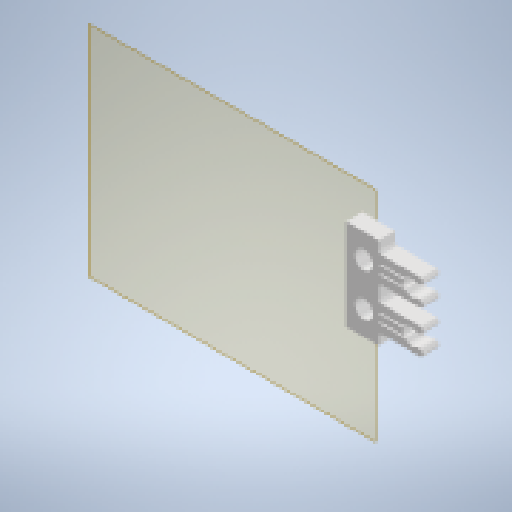
# Autodesk Inventor part: Fuse holdere
Saved by Autodesk Inventor 2024 (Build 280153000, 153)
## iProperties
Created: 2024-03-29
Part Number: Fuse holdere
Material: Generic
Document SubType Name: Modeling
Designer: jens1
Density: 1 g/cm^3
Appearance: Default
Author: jens1
Autodesk Inventor part; units mm, degrees
ref_plane "YZ Plane" through (0, 0, 0) normal (1, 0, 0) x (0, 1, 0)
ref_plane "XZ Plane" through (0, 0, 0) normal (0, 1, 0) x (-1, 0, 0)
ref_plane "XY Plane" through (0, 0, 0) normal (0, 0, 1) x (1, 0, 0)
ref_plane "Work Plane1" through (373.0741, 421.919, 355.2069) normal (0, 0, 1) x (1, 0, 0)
sketch "Sketch1" plane through (373.0741, 421.919, 355.2069) normal (0, 0, 1) x (1, 0, 0)
  line L0 (-40, 30.5) -> (-40, -30.5) projected
  line L1 (-40, -30.5) -> (45, -30.5) projected
  circle A0 centre (5.1305, -24.4679) radius 3.2 projected
  circle A1 centre (-24.4679, -5.1305) radius 3.2 projected
  circle A2 centre (-5.1305, 24.4679) radius 3.2 projected
  circle A3 centre (24.4679, 5.1305) radius 3.2 projected
  circle A4 centre (0, 0) radius 16.75 projected
  line L2 (40, 25.5) -> (50, 25.5)
  line L3 (50, 25.5) -> (50, -25.5)
  line L4 (50, -25.5) -> (40, -25.5)
  line L5 (40, -25.5) -> (40, 25.5)
  circle A5 centre (60, 18) radius 2.25
  circle A6 centre (60, 18) radius 2.5
  line L6 (50, 19) -> (57.7087, 19)
  line L7 (57.7087, 19) -> (57.7087, 17)
  line L8 (57.7087, 17) -> (50, 17)
  line L9 (50, 17) -> (50, 19)
  line L10 (50, 19.5) -> (58.3229, 19.5)
  line L11 (57.7087, 18) -> (50, 18)
  line L12 (58.3229, 16.5) -> (50, 16.5)
  line L13 (62.6125, 22) -> (50, 22)
  line L14 (50, 14) -> (62.6125, 14)
  line L15 (63.5021, 20.5433) -> (62.2478, 18.1)
  line L16 (63.5021, 15.4567) -> (62.2478, 17.9)
  arc A7 (63.5021, 20.5433) -> (62.6125, 22) centre (62.6125, 21) ccw
  arc A8 (62.6125, 14) -> (63.5021, 15.4567) centre (62.6125, 15) ccw
  line L17 (50, 11.5) -> (40, 11.5)
  circle A9 centre (60, 5) radius 2.25
  circle A10 centre (60, 5) radius 2.5
  line L18 (50, 4) -> (57.7087, 4)
  line L19 (57.7087, 6) -> (50, 6)
  line L20 (50, 3.5) -> (58.3229, 3.5)
  line L21 (58.3229, 6.5) -> (50, 6.5)
  line L22 (62.6125, 1) -> (50, 1)
  line L23 (50, 9) -> (62.6125, 9)
  line L24 (63.5021, 2.4567) -> (62.2478, 4.9)
  line L25 (63.5021, 7.5433) -> (62.2478, 5.1)
  arc A11 (62.6125, 1) -> (63.5021, 2.4567) centre (62.6125, 2) ccw
  arc A12 (63.5021, 7.5433) -> (62.6125, 9) centre (62.6125, 8) ccw
  line L26 (40, 25.5) -> (50, 25.5)
  line L27 (50, 25.5) -> (50, -2.5)
  line L28 (50, -2.5) -> (40, -2.5)
  line L29 (40, -2.5) -> (40, 25.5)
  circle A13 centre (45.3451, 5) radius 2.5 projected
  circle A14 centre (45, -8) radius 2.5 projected
  circle A15 centre (45.3451, 18) radius 2.5 projected
  circle A16 centre (45, -21) radius 2.5 projected
  arc A17 (45, -30.5) -> (50, -25.5) centre (45, -25.5) ccw projected
  line L30 (50, 25.5) -> (50, -25.5) projected
  arc A18 (50, 25.5) -> (45, 30.5) centre (45, 25.5) ccw projected
  line L31 (-40, 30.5) -> (45, 30.5) projected
  point P0 (-373.0741, -421.919)
  point P1 (40, 30.5)
  point P2 (53.8544, 18)
  point P3 (64.25, 22)
  point P4 (64.25, 14)
  point P5 (50, 1)
  point P6 (62.2478, 4.9)
  point P7 (50, 3.5)
  point P8 (50, 4)
  point P9 (50, 6)
  point P10 (50, 6.5)
  point P11 (50, 9)
  point P12 (50, 17)
  point P13 (62.2478, 18.1)
  point P14 (40, -2.5)
  point P15 (62.4505, 17.5051)
  point P16 (58, 16.5)
  point P17 (50, 16.5)
  point P18 (50, 14)
  point P19 (50, 22)
  point P20 (50, 19.5)
  point P21 (58, 19.5)
  point P22 (62.4505, 18.4949)
  point P23 (50, 9)
  point P24 (50, 6.5)
  point P25 (58, 6.5)
  point P26 (62.4505, 5.4949)
  point P27 (50, 17)
  point P28 (50, 19)
  point P29 (62.4505, 4.5051)
  point P30 (58, 3.5)
  point P31 (50, 3.5)
  point P32 (50, 1)
  point P33 (50, 6)
  point P34 (50, 4)
  point P35 (40, -2.5)
  dimension "d1" = 5
  dimension "d4" = 4.5
  dimension "d5" = 5
  dimension "d6" = 10
  dimension "d7" = 2
  dimension "d8" = 1
  dimension "d9" = 1.5
  dimension "d10" = 1.5
  dimension "d11" = 2.5
  dimension "d12" = 2.5
  dimension "d13" = 14.25
  dimension "d14" = 14.25
  dimension "d15" = 0.2
  dimension "d16" = 0
  dimension "d17" = 0.1
  dimension "d18" = 1
  dimension "d19" = 3.5
  dimension "d20" = 6.5
  dimension "d21" = 3.5
  constraints: 54 end point, 20 symmetric about line, 18 point on circle, 11 parallel, 8 centre point, 5 point on line, 4 horizontal, 4 tangent, 3 midpoint, 2 coincident, 2 perpendicular, 1 equal radius, 1 vertical, 15 other
  measures "d1" distance between parallel lines of L1 L4
  measures "d4" diameter of A5
  measures "d5" diameter of A6
  measures "d7" distance of L6.end L7.end
  measures "d8" distance between parallel lines of L8 L11
  measures "d9" distance from line of L10 point (53.854, 18)
  measures "d10" distance between parallel lines of L12 L11
  measures "d11" distance between parallel lines of L10 L13
  measures "d12" distance between parallel lines of L12 L14
  measures "d13" distance of point (64.25, 22) L13.end
  measures "d14" distance of L14.start point (64.25, 14)
  measures "d15" distance of L16.end L15.end
  measures "d16" horizontal distance of L15.end L16.end
  measures "d17" vertical distance of A5.centre L16.end
  measures "d18" radius of A7
  measures "d19" distance between parallel lines of L2 L13
  measures "d20" distance from line of A5.centre L17
  measures "d21" distance between parallel lines of L22 L28
extrude "Extrusion1" add sketch "Sketch1" along normal blind 5 contours L3 L17 L5 L2 | L13 A7 L15 A6 L10 L3 | L28 L5 L17 L3 | L3 L20 A10 L24 A11 L22 | L6 A6 L11 L3 | L3 L12 A6 L16 A8 L14 | L23 A12 L25 A10 L21 L3 | L11 A6 L8 L3 | L3 L19 A10 L18 | A13 | A15
fillet "Fillet1" radius 2 4 edges at (435.5246, 440.414, 357.7069) (435.5246, 439.4241, 357.7069) (435.5246, 427.414, 357.7069) (435.5246, 426.4241, 357.7069)
fillet "Fillet2" radius 1 8 edges at (423.0741, 441.419, 357.7069) (423.0741, 438.419, 357.7069) (423.0741, 443.919, 357.7069) (423.0741, 435.919, 357.7069) (423.0741, 430.919, 357.7069) (423.0741, 428.419, 357.7069) (423.0741, 425.419, 357.7069) (423.0741, 422.919, 357.7069)
sketch "Sketch2" plane through (373.0741, 421.919, 360.2069) normal (0, 0, 1) x (1, 0, 0)
  line L0 (58, 3.5) -> (50.866, 3.5) projected
  line L1 (50, 4) -> (57.7087, 4) projected
  arc A0 (57.7087, 6) -> (57.7087, 4) centre (60, 5) ccw projected
  line L2 (57.7087, 6) -> (50, 6) projected
  line L3 (50.866, 6.5) -> (58, 6.5) projected
  arc A1 (63.5021, 7.5433) -> (62.6125, 9) centre (62.6125, 8) ccw projected
  line L4 (62.6125, 9) -> (51, 9) projected
  line L5 (50, 10) -> (50, 13) projected
  line L6 (51, 14) -> (62.6125, 14) projected
  arc A2 (62.6125, 14) -> (63.5021, 15.4567) centre (62.6125, 15) ccw projected
  line L7 (58, 16.5) -> (50.866, 16.5) projected
  line L8 (50, 17) -> (57.7087, 17) projected
  arc A3 (57.7087, 19) -> (57.7087, 17) centre (60, 18) ccw projected
  line L9 (57.7087, 19) -> (50, 19) projected
  line L10 (50.866, 19.5) -> (58, 19.5) projected
  arc A4 (63.5021, 20.5433) -> (62.6125, 22) centre (62.6125, 21) ccw projected
  line L11 (62.6125, 22) -> (51, 22) projected
  line L12 (50, 25.5) -> (40, 25.5) projected
  line L13 (51, 1) -> (62.6125, 1) projected
  arc A5 (62.6125, 1) -> (63.5021, 2.4567) centre (62.6125, 2) ccw projected
  arc A6 (58, 3.5) -> (61.1705, 2.791) centre (60, 5) ccw projected
  arc A7 (61.1705, 7.209) -> (58, 6.5) centre (60, 5) ccw projected
  arc A8 (58, 16.5) -> (61.1705, 15.791) centre (60, 18) ccw projected
  arc A9 (61.1705, 20.209) -> (58, 19.5) centre (60, 18) ccw projected
  line L14 (40, 25.5) -> (40, -2.5) projected
  arc A10 (50, 10) -> (51, 9) centre (51, 10) ccw projected
  arc A11 (51, 14) -> (50, 13) centre (51, 13) ccw projected
  arc A12 (50, 17) -> (50.866, 16.5) centre (50.866, 17.5) ccw projected
  arc A13 (50.866, 19.5) -> (50, 19) centre (50.866, 18.5) ccw projected
  arc A14 (50, 23) -> (51, 22) centre (51, 23) ccw projected
  line L15 (50, 23) -> (50, 25.5) projected
  line L16 (40, -2.5) -> (50, -2.5) projected
  line L17 (50, -2.5) -> (50, 0) projected
  arc A15 (51, 1) -> (50, 0) centre (51, 0) ccw projected
  arc A16 (50, 4) -> (50.866, 3.5) centre (50.866, 4.5) ccw projected
  arc A17 (50.866, 6.5) -> (50, 6) centre (50.866, 5.5) ccw projected
  arc A18 (63.5021, 2.4567) -> (61.1705, 2.791) centre (62.107, 1.0237) ccw projected
  arc A19 (61.1705, 7.209) -> (63.5021, 7.5433) centre (62.107, 8.9763) ccw projected
  arc A20 (63.5021, 15.4567) -> (61.1705, 15.791) centre (62.107, 14.0237) ccw projected
  arc A21 (61.1705, 20.209) -> (63.5021, 20.5433) centre (62.107, 21.9763) ccw projected
  point P0 (-373.0741, -421.919)
  point P1 (45.3451, 18)
  point P2 (45.3451, 5)
  dimension "d26" = 0
  dimension "d27" = 13
  dimension "d28" = 7.5
  measures "d26" horizontal distance of point (45.345, 5) point (45.345, 18)
  measures "d27" distance of point (45.345, 18) point (45.345, 5)
  measures "d28" distance from line of L12 point (45.345, 18)
hole "Hole1" at (418.4192, 439.919, 360.2069) at (418.4192, 426.919, 360.2069) direction (0, 0, -1) diameter 5.5 end through all
sketch "Sketch3" plane through (373.0741, 421.919, 355.2069) normal (0, 0, 1) x (1, 0, 0)
  line L0 (68.3936, 26.3924) -> (78.3936, 26.3924)
  line L1 (78.3936, 26.3924) -> (78.3936, -1.6076)
  line L2 (78.3936, -1.6076) -> (68.3936, -1.6076)
  line L3 (68.3936, -1.6076) -> (68.3936, 26.3924)
  line L4 (78.3936, 26.3924) -> (68.3936, 26.3924)
  line L5 (68.3936, 26.3924) -> (68.3936, 12.3924)
  line L6 (68.3936, 12.3924) -> (78.3936, 12.3924)
  line L7 (78.3936, 12.3924) -> (78.3936, 26.3924)
  line L8 (92.6436, 14.3924) -> (78.3936, 14.3924)
  line L9 (78.3936, 14.3924) -> (78.3936, 14.5958)
  line L10 (78.3936, 19.3924) -> (86.1023, 19.3924)
  line L11 (86.1023, 19.3924) -> (86.1023, 17.3924)
  line L12 (86.1023, 17.3924) -> (78.3936, 17.3924)
  line L13 (78.3936, 17.3924) -> (78.3936, 19.3924)
  circle A0 centre (88.3936, 18.3924) radius 2.25
  circle A1 centre (88.3936, 18.3924) radius 2.5
  line L14 (91.6425, 23.6467) -> (90.6413, 18.4924)
  line L15 (92.6436, 14.3924) -> (90.6413, 18.2924)
  line L16 (78.3936, 16.8924) -> (86.3936, 16.8924)
  line L17 (78.1639, 19.8924) -> (86.3936, 19.8924)
  line L18 (78.3936, 23.6467) -> (91.6425, 23.6467)
  point P0 (-373.0741, -421.919)
  point P1 (73.3936, 26.3924)
  point P2 (82.2479, 17.3924)
  dimension "d36" = 10
  dimension "d37" = 28
  dimension "d38" = 14
  dimension "d44" = 2
  dimension "d45" = 4.5
  dimension "d46" = 5
  dimension "d47" = 1
  dimension "d48" = 10
  dimension "d49" = 0.2
  dimension "d50" = 0.1
  dimension "d51" = 14.25
  dimension "d53" = 2.5
  dimension "d54" = 0.5
  dimension "d55" = 0.5
  dimension "d57" = 90
  constraints: 38 end point, 7 parallel, 5 point on circle, 4 midpoint, 3 horizontal, 3 perpendicular, 3 point on line, 2 centre point, 1 coincident
  measures "d36" distance of L1.end L2.end
  measures "d37" distance of L0.end L1.end
  measures "d38" distance from line of point (73.394, 26.392) L6
  measures "d44" distance from line of point (82.248, 17.392) L10
  measures "d45" diameter of A0
  measures "d46" diameter of A1
  measures "d47" distance from line of A0.centre L10
  measures "d48" distance from line of L1 A0.centre
  measures "d49" distance of L14.end L15.end
  measures "d50" vertical distance of A0.centre L15.end
  measures "d51" distance of L8.start L8.end
  measures "d53" distance between parallel lines of L8 L16
  measures "d54" distance between parallel lines of L12 L16
  measures "d55" distance between parallel lines of L10 L17
  measures "d57" angle of L1 L18
equation "\"d8\" = 0.5 * d7"
equation "\"d10\" = d9"
equation "\"d12\" = d11"
equation "\"d14\" = d13"
equation "\"d17\" = 0.5 * d15"
equation "\"d38\" = 0.5 * d37"
equation "\"d51\" = d41"
equation "\"d41\" = 14.25"
body "Solid1"
